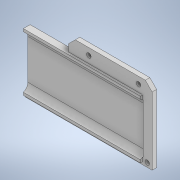
# Autodesk Inventor part: hdmi_base_plate
Saved by Autodesk Inventor 2021 (Build 250183000, 183)
## iProperties
Created: 2026-02-14
Part Number: hdmi_base_plate
Material: Generic
Document SubType Name: Modeling
Designer: Toby
Density: 1 g/cm^3
Appearance: Default
Author: Toby
Autodesk Inventor part; units mm, degrees
ref_plane "YZ Plane" through (0, 0, 0) normal (1, 0, 0) x (0, 1, 0)
ref_plane "XZ Plane" through (0, 0, 0) normal (0, 1, 0) x (-1, 0, 0)
ref_plane "XY Plane" through (0, 0, 0) normal (0, 0, 1) x (1, 0, 0)
sketch "Sketch1" plane through (0, 0, 0) normal (0, 0, 1) x (1, 0, 0)
  line L0 (-28, 16.5) -> (28, 16.5)
  line L1 (28, 16.5) -> (28, -16.5)
  line L2 (28, -16.5) -> (-28, -16.5)
  line L3 (-28, -16.5) -> (-28, 16.5)
  point P0 (0, 0)
  dimension "d0" = 33
  dimension "d1" = 56
  dimension "d2" = 16.5
  dimension "d3" = 28
  constraints: 8 end point, 2 parallel, 1 horizontal, 1 perpendicular
  measures "d0" distance of L2.end L0.start
  measures "d1" distance of L0.start L0.end
  measures "d2" distance from line of point (0, 0) L0
  measures "d3" distance from line of point (0, 0) L3
extrude "Extrusion1" add sketch "Sketch1" along normal blind 2
sketch "Sketch2" plane through (0, 0, 2) normal (0, 0, 1) x (1, 0, 0)
  line L0 (-28, 16.5) -> (-28, -16.5) projected
  line L1 (-28, -16.5) -> (28, -16.5) projected
  circle A0 centre (0, 13.5) radius 1
  circle A1 centre (22, 13.5) radius 1
  point P0 (0, 0)
  dimension "d6" = 28
  dimension "d7" = 30
  dimension "d8" = 50
  dimension "d9" = 30
  dimension "d10" = 2
  dimension "d11" = 2
  constraints: 2 centre point, 2 coincident
  measures "d6" distance from line of L0 point (0, 13.5)
  measures "d7" distance from line of L1 point (0, 13.5)
  measures "d8" distance from line of L0 point (22, 13.5)
  measures "d9" distance from line of L1 point (22, 13.5)
  measures "d10" diameter of A0
  measures "d11" diameter of A1
extrude "Extrusion2" cut sketch "Sketch2" against normal blind 2
sketch "Sketch3" plane through (0, 0, 2) normal (0, 0, 1) x (1, 0, 0)
  line L0 (-28, 16.5) -> (-28, -16.5) projected
  line L1 (-28, 11.5) -> (24, 11.5)
  line L2 (24, 11.5) -> (24, -14.1)
  line L3 (24, -14.1) -> (-28, -14.1)
  line L4 (-28, -14.1) -> (-28, 11.5)
  line L5 (-28, -16.5) -> (28, -16.5) projected
  line L6 (-28, 11.5) -> (24, 11.5)
  line L7 (24, 11.5) -> (24, 9.1)
  line L8 (24, 9.1) -> (-28, 9.1)
  line L9 (-28, 9.1) -> (-28, 11.5)
  point P0 (0, 0)
  point P1 (-28, 9.1)
  dimension "d14" = 2.4
  dimension "d15" = 28
  dimension "d16" = 2.4
  dimension "d17" = 52
  constraints: 16 end point, 4 parallel, 2 horizontal, 2 perpendicular, 2 point on line
  measures "d14" distance between parallel lines of L5 L3
  measures "d15" distance between parallel lines of L5 L1
  measures "d16" distance between parallel lines of L8 L1
  measures "d17" distance between parallel lines of L0 L2
extrude "Extrusion3" cut sketch "Sketch3" against normal blind 1 contours L8 L2 L3 L0
sketch "Sketch4" plane through (0, 0, 2) normal (0, 0, 1) x (1, 0, 0)
  line L0 (-28, -14.1) -> (-28, 9.1) projected
  line L1 (-28, -16.5) -> (28, -16.5) projected
  circle A0 centre (25.87, -14.63) radius 1
  point P0 (0, 0)
  dimension "d23" = 53.87
  dimension "d24" = 1.87
  dimension "d25" = 2
  constraints: 1 centre point, 1 coincident
  measures "d23" distance from line of L0 point (25.87, -14.63)
  measures "d24" distance from line of L1 point (25.87, -14.63)
  measures "d25" diameter of A0
extrude "Extrusion4" cut sketch "Sketch4" against normal blind 2
chamfer "Chamfer2" distance 3 angle 45 1 edges at (28, 16.5, 1)
sketch "Sketch8" plane through (0, 0, 2) normal (0, 0, 1) x (1, 0, 0)
  line L0 (25, 16.5) -> (-28, 16.5) projected
  line L1 (-28, 16.5) -> (-9, 16.5)
  line L2 (-9, 16.5) -> (-9, 10.3)
  line L3 (-9, 10.3) -> (-28, 10.3)
  line L4 (-28, 10.3) -> (-28, 16.5)
  line L5 (-28, 9.1) -> (24, 9.1) projected
  point P0 (0, 0)
  dimension "d40" = 19
  dimension "d41" = 1.2
  constraints: 8 end point, 2 parallel, 1 horizontal, 1 perpendicular
  measures "d40" distance of L2.end L3.end
  measures "d41" distance between parallel lines of L3 L5
extrude "Extrusion7" cut sketch "Sketch8" against normal blind 2
chamfer "Chamfer4" distance 3 angle 45 1 edges at (-9, 16.5, 1)
sketch "Sketch9" plane through (0, 0, 2) normal (0, 0, 1) x (1, 0, 0)
  line L0 (-28, 10.3) -> (-9, 10.3) projected
  line L1 (-28, 9.1) -> (24, 9.1) projected
  line L2 (-28, 10.3) -> (24, 10.3)
  line L3 (24, 10.3) -> (24, 9.1)
  line L4 (24, 9.1) -> (-28, 9.1)
  line L5 (-28, 9.1) -> (-28, 10.3)
  line L6 (24, -14.1) -> (-28, -14.1) projected
  line L7 (-28, -14.1) -> (24, -14.1)
  line L8 (24, -14.1) -> (24, -15.3)
  line L9 (24, -15.3) -> (-28, -15.3)
  line L10 (-28, -15.3) -> (-28, -14.1)
  line L11 (24, 9.1) -> (24, -14.1) projected
  point P0 (0, 0)
  dimension "d47" = 1.2
  constraints: 16 end point, 4 parallel, 2 horizontal, 2 perpendicular, 1 collinear
  measures "d47" distance between parallel lines of L6 L9
extrude "Extrusion8" add sketch "Sketch9" along normal blind 1
fillet "Fillet1" radius 3 2 edges at (-2, 9.1, 1) (-2, -14.1, 1)
sketch "Sketch10" plane through (0, 0, 3) normal (0, 0, 1) x (1, 0, 0)
  line L0 (24, 9.1) -> (24, 10.3) projected
  line L1 (-28, -15.3) -> (24, -15.3) projected
  line L2 (24, 10.3) -> (23.8, 10.3)
  line L3 (23.8, 10.3) -> (23.8, -15.3)
  line L4 (23.8, -15.3) -> (24, -15.3)
  line L5 (24, -15.3) -> (24, 10.3)
  point P0 (0, 0)
  dimension "d51" = 0.2
  constraints: 8 end point, 2 parallel, 1 horizontal, 1 perpendicular, 1 point on line
  measures "d51" distance between parallel lines of L5 L3
extrude "Extrusion9" cut sketch "Sketch10" against normal blind 1
body "Solid1"
